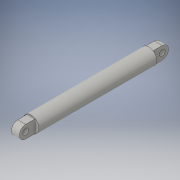
# Autodesk Inventor part: body to wheel hub connectors (19 in)
Saved by Autodesk Inventor 2016 (Build 200138000, 138)
## iProperties
Created: 2017-06-26
Part Number: body to wheel hub connectors (19 in)
Material: Generic
Document SubType Name: Modeling
Designer: andon
Density: 1 g/cm^3
Appearance: Default
Author: andon
Autodesk Inventor part; units mm, degrees
ref_plane "YZ Plane" through (0, 0, 0) normal (1, 0, 0) x (0, 1, 0)
ref_plane "XZ Plane" through (0, 0, 0) normal (0, 1, 0) x (-1, 0, 0)
ref_plane "XY Plane" through (0, 0, 0) normal (0, 0, 1) x (1, 0, 0)
sketch "Sketch1" plane through (0, 0, 0) normal (0, 0, 1) x (1, 0, 0)
  circle A0 centre (0, 0) radius 25.4
  dimension "d0" = 50.8
  constraints: 1 centre point, 1 coincident
  measures "d0" diameter of A0
extrude "Extrusion1" add sketch "Sketch1" along normal mid plane 381
sketch "Sketch4" plane through (0, 0, 190.5) normal (0, 0, 1) x (1, 0, 0)
  line L0 (-12.7, 20.6375) -> (12.7, 20.6375)
  line L1 (12.7, 20.6375) -> (12.7, -20.6375)
  line L2 (12.7, -20.6375) -> (-12.7, -20.6375)
  line L3 (-12.7, -20.6375) -> (-12.7, 20.6375)
  line L4 (-12.7, 20.6375) -> (12.7, -20.6375) construction
  line L5 (12.7, 20.6375) -> (-12.7, -20.6375) construction
  point P0 (0, 0)
  dimension "d15" = 25.4
  dimension "d16" = 41.275
  constraints: 12 end point, 2 midpoint, 2 parallel, 1 horizontal, 1 perpendicular
  measures "d15" distance between parallel lines of L1 L3
  measures "d16" distance between parallel lines of L2 L0
extrude "Extrusion4" add sketch "Sketch4" along normal blind 50.8
fillet "Fillet2" radius 20.6375 2 edges at (0, 20.6375, 241.3) (0, -20.6375, 241.3)
sketch "Sketch5" plane through (12.7, -20.6375, 190.5) normal (1, 0, 0) x (0, 0, -1)
  arc A0 (-30.1625, 41.275) -> (-30.1625, 0) centre (-30.1625, 20.6375) ccw projected
  circle A1 centre (-30.1625, 20.6375) radius 9.525
  point P0 (190.5, 20.6375)
  constraints: 1 centre point, 1 coincident
extrude "Extrusion5" cut sketch "Sketch5" against normal blind 50.8
mirror "Mirror1" about plane through (0, 0, 0) normal (0, 0, 1) of "Extrusion4", "Fillet2", "Extrusion5"
body "Solid1"
